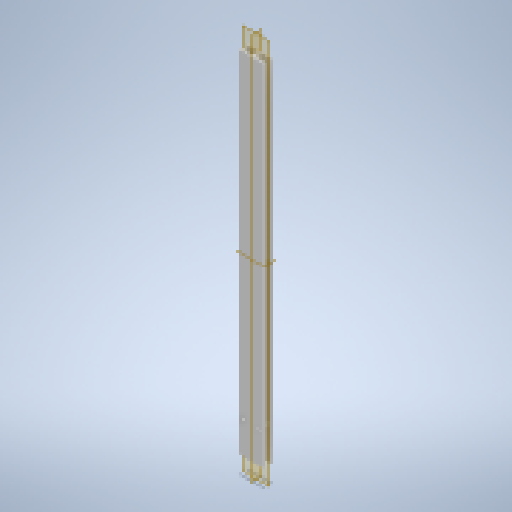
# Autodesk Inventor part: Алюминиевый профиль
Saved by Autodesk Inventor 2023.2 (Build 272271030, 271C)
## iProperties
Created: 2024-03-12
Part Number: Алюминиевый профиль
Material: Типовые
Document SubType Name: Modeling
Designer: I9232
Density: 1 g/cm^3
Appearance: По умолчанию
Author: I9232
Autodesk Inventor part; units mm, degrees
sketch "Эскиз1" plane through (0, 0, 0) normal (0, 1, 0) x (-1, 0, 0)
  line L0 (0.8, -3.3) -> (0.8, 3.3)
  line L1 (-0.8, -3.3) -> (-0.8, 3.3)
  line L2 (-17.675, 0) -> (17.675, 0) construction
  line L3 (0.8, 0) -> (-0.8, 0) construction
  line L4 (0, -4.62) -> (0, 4.62)
  line L5 (12.625, -3.3) -> (0.8, -3.3)
  line L6 (-0.8, -3.3) -> (-12.625, -3.3)
  line L7 (12.625, 3.3) -> (0.8, 3.3)
  line L8 (-0.8, 3.3) -> (-12.625, 3.3)
  line L9 (12.625, -4.9) -> (-12.625, -4.9)
  line L10 (12.625, 4.9) -> (-12.625, 4.9)
  line L11 (12.625, -3.3) -> (12.625, -4.9)
  line L12 (-12.625, -3.3) -> (-12.625, -4.9)
  line L13 (-12.625, 4.9) -> (-12.625, 3.3)
  line L14 (12.625, 4.9) -> (12.625, 3.3)
  point P0 (0, 0)
  dimension "d0" = 1.6
  dimension "d1" = 6.6
  dimension "d2" = 25.25
  dimension "d3" = 1.6
  dimension "d4" = 1.6
  constraints: 28 end point, 4 horizontal, 3 midpoint, 3 parallel, 3 vertical, 2 collinear, 2 point on line, 2 symmetric about line
  measures "d0" distance between parallel lines of L1 L0
  measures "d1" distance of L0.end L0.start
  measures "d2" distance of L5.start L6.end
  measures "d3" distance between parallel lines of L9 L6
  measures "d4" distance between parallel lines of L10 L8
extrude "Выдавливание1" add sketch "Эскиз1" along normal mid plane 360
sketch "Эскиз4" plane through (12.625, 180, -4.9) normal (0, 0, -1) x (-1, 0, 0)
  circle A0 centre (4.625, -327) radius 1.5 projected
  circle A1 centre (20.625, -327) radius 1.5 projected
  point P0 (12.625, -180)
extrude "Выдавливание4" cut sketch "Эскиз4" against normal up to surface (1.6 mm away)
sketch "Эскиз5" plane through (-12.625, 180, 4.9) normal (0, 0, 1) x (1, 0, 0)
  circle A0 centre (4.625, -327) radius 1.5 projected
  circle A1 centre (20.625, -327) radius 1.5 projected
  point P0 (12.625, -180)
extrude "Выдавливание5" cut sketch "Эскиз5" against normal up to surface (1.6 mm away)
